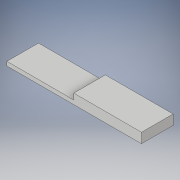
# Autodesk Inventor part: Mesh Test
Saved by Autodesk Inventor 2017.3 (Build 213256000, 256)
## iProperties
Created: 2019-02-15
Part Number: Mesh Test
Material: Generic
Document SubType Name: Modeling
Designer: LSabe
Density: 1 g/cm^3
Appearance: Default
Author: LSabe
Autodesk Inventor part; units mm, degrees
ref_plane "YZ Plane" through (0, 0, 0) normal (1, 0, 0) x (0, 1, 0)
ref_plane "XZ Plane" through (0, 0, 0) normal (0, 1, 0) x (-1, 0, 0)
ref_plane "XY Plane" through (0, 0, 0) normal (0, 0, 1) x (1, 0, 0)
sketch "Sketch1" plane through (0, 0, 0) normal (0, 0, 1) x (1, 0, 0)
  line L0 (38.354, 0) -> (76.2, 0)
  line L1 (76.2, 0) -> (76.2, 2.794)
  line L2 (76.2, 2.794) -> (57.15, 2.794)
  line L3 (57.15, 1.143) -> (57.15, 2.794)
  line L4 (38.354, 1.143) -> (57.15, 1.143)
  line L5 (38.354, 1.143) -> (38.354, 0)
  point P0 (0, 0)
  constraints: 12 end point, 2 perpendicular, 1 horizontal, 1 parallel
extrude "Extrusion1" add sketch "Sketch1" along normal blind 8.89
body "Solid1"
